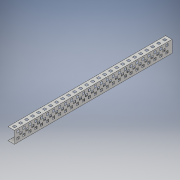
# Autodesk Inventor part: 1sqr x 2sqr x 1sqr metal frame (large)
Saved by Autodesk Inventor 2018 (Build 220112000, 112)
## iProperties
Created: 2018-11-08
Part Number: 1sqr x 2sqr x 1sqr metal frame (large)
Material: Generic
Document SubType Name: Modeling
Designer: USER
Density: 1 g/cm^3
Appearance: Default
Author: USER
Autodesk Inventor part; units mm, degrees
ref_plane "YZ Plane" through (0, 0, 0) normal (1, 0, 0) x (0, 1, 0)
ref_plane "XZ Plane" through (0, 0, 0) normal (0, 1, 0) x (-1, 0, 0)
ref_plane "XY Plane" through (0, 0, 0) normal (0, 0, 1) x (1, 0, 0)
sketch "Sketch1" plane through (0, 0, 0) normal (1, 0, 0) x (0, 1, 0)
  line L0 (0, 0) -> (-24, 0)
  line L1 (-24, 0) -> (-24, -315)
  line L2 (-24, -315) -> (0, -315)
  line L3 (0, -315) -> (0, 0)
  dimension "d0" = 24
  dimension "d1" = 315
  constraints: 8 end point, 2 parallel, 1 horizontal, 1 perpendicular
  measures "d0" distance of L2.end L1.end
  measures "d1" distance of L1.end L0.end
sketch "Sketch2" plane through (0, 0, 0) normal (0, 1, 0) x (-1, 0, 0)
  line L0 (0, 0) -> (13, 0)
  line L1 (13, 0) -> (13, -315)
  line L2 (13, -315) -> (0, -315)
  line L3 (0, -315) -> (0, 0)
  dimension "d2" = 13
  dimension "d3" = 315
  constraints: 8 end point, 2 parallel, 1 horizontal, 1 perpendicular
  measures "d2" distance of L1.end L2.end
  measures "d3" distance of L0.end L1.end
extrude "Extrusion1" add sketch "Sketch2" along normal blind 0.1
extrude "Extrusion2" add sketch "Sketch1" along normal blind 0.1 separate body
sketch "Sketch3" plane through (0, -24, -315) normal (0, -1, 0) x (1, 0, 0)
  line L0 (-13, 315) -> (0, 315) projected
  line L1 (0, 315) -> (-13, 315)
  line L2 (-13, 315) -> (-13, 0)
  line L3 (-13, 0) -> (0, 0)
  line L4 (0, 0) -> (0, 315)
  dimension "d8" = 13
  dimension "d9" = 315
  constraints: 8 end point, 2 parallel, 1 horizontal, 1 perpendicular
  measures "d8" distance of L3.end L2.end
  measures "d9" distance of L2.end L1.end
extrude "Extrusion3" add sketch "Sketch3" along normal blind 0.1 separate body
sketch "Sketch4" plane through (0, 0.1, 0) normal (0, 1, 0) x (1, 0, 0)
  line L0 (-8.9107, 4.7757) -> (-4.3387, 4.7757)
  line L1 (-4.3387, 4.7757) -> (-4.3387, 9.3477)
  line L2 (-4.3387, 9.3477) -> (-8.9107, 9.3477)
  line L3 (-8.9107, 9.3477) -> (-8.9107, 4.7757)
  line L4 (-8.9107, 21.3477) -> (-8.9107, 16.7757)
  line L5 (-8.9107, 16.7757) -> (-4.3387, 16.7757)
  line L6 (-4.3387, 16.7757) -> (-4.3387, 21.3477)
  line L7 (-4.3387, 21.3477) -> (-8.9107, 21.3477)
  line L8 (-8.9107, 33.3477) -> (-8.9107, 28.7757)
  line L9 (-8.9107, 28.7757) -> (-4.3387, 28.7757)
  line L10 (-4.3387, 28.7757) -> (-4.3387, 33.3477)
  line L11 (-4.3387, 33.3477) -> (-8.9107, 33.3477)
  line L12 (-8.9107, 45.3477) -> (-8.9107, 40.7757)
  line L13 (-8.9107, 40.7757) -> (-4.3387, 40.7757)
  line L14 (-4.3387, 40.7757) -> (-4.3387, 45.3477)
  line L15 (-4.3387, 45.3477) -> (-8.9107, 45.3477)
  line L16 (-8.9107, 57.3477) -> (-8.9107, 52.7757)
  line L17 (-8.9107, 52.7757) -> (-4.3387, 52.7757)
  line L18 (-4.3387, 52.7757) -> (-4.3387, 57.3477)
  line L19 (-4.3387, 57.3477) -> (-8.9107, 57.3477)
  line L20 (-8.9107, 69.3477) -> (-8.9107, 64.7757)
  line L21 (-8.9107, 64.7757) -> (-4.3387, 64.7757)
  line L22 (-4.3387, 64.7757) -> (-4.3387, 69.3477)
  line L23 (-4.3387, 69.3477) -> (-8.9107, 69.3477)
  line L24 (-8.9107, 81.3477) -> (-8.9107, 76.7757)
  line L25 (-8.9107, 76.7757) -> (-4.3387, 76.7757)
  line L26 (-4.3387, 76.7757) -> (-4.3387, 81.3477)
  line L27 (-4.3387, 81.3477) -> (-8.9107, 81.3477)
  line L28 (-8.9107, 93.3477) -> (-8.9107, 88.7757)
  line L29 (-8.9107, 88.7757) -> (-4.3387, 88.7757)
  line L30 (-4.3387, 88.7757) -> (-4.3387, 93.3477)
  line L31 (-4.3387, 93.3477) -> (-8.9107, 93.3477)
  line L32 (-8.9107, 105.3477) -> (-8.9107, 100.7757)
  line L33 (-8.9107, 100.7757) -> (-4.3387, 100.7757)
  line L34 (-4.3387, 100.7757) -> (-4.3387, 105.3477)
  line L35 (-4.3387, 105.3477) -> (-8.9107, 105.3477)
  line L36 (-8.9107, 117.3477) -> (-8.9107, 112.7757)
  line L37 (-8.9107, 112.7757) -> (-4.3387, 112.7757)
  line L38 (-4.3387, 112.7757) -> (-4.3387, 117.3477)
  line L39 (-4.3387, 117.3477) -> (-8.9107, 117.3477)
  line L40 (-8.9107, 129.3477) -> (-8.9107, 124.7757)
  line L41 (-8.9107, 124.7757) -> (-4.3387, 124.7757)
  line L42 (-4.3387, 124.7757) -> (-4.3387, 129.3477)
  line L43 (-4.3387, 129.3477) -> (-8.9107, 129.3477)
  line L44 (-8.9107, 141.3477) -> (-8.9107, 136.7757)
  line L45 (-8.9107, 136.7757) -> (-4.3387, 136.7757)
  line L46 (-4.3387, 136.7757) -> (-4.3387, 141.3477)
  line L47 (-4.3387, 141.3477) -> (-8.9107, 141.3477)
  line L48 (-8.9107, 153.3477) -> (-8.9107, 148.7757)
  line L49 (-8.9107, 148.7757) -> (-4.3387, 148.7757)
  line L50 (-4.3387, 148.7757) -> (-4.3387, 153.3477)
  line L51 (-4.3387, 153.3477) -> (-8.9107, 153.3477)
  line L52 (-8.9107, 165.3477) -> (-8.9107, 160.7757)
  line L53 (-8.9107, 160.7757) -> (-4.3387, 160.7757)
  line L54 (-4.3387, 160.7757) -> (-4.3387, 165.3477)
  line L55 (-4.3387, 165.3477) -> (-8.9107, 165.3477)
  line L56 (-8.9107, 177.3477) -> (-8.9107, 172.7757)
  line L57 (-8.9107, 172.7757) -> (-4.3387, 172.7757)
  line L58 (-4.3387, 172.7757) -> (-4.3387, 177.3477)
  line L59 (-4.3387, 177.3477) -> (-8.9107, 177.3477)
  line L60 (-8.9107, 189.3477) -> (-8.9107, 184.7757)
  line L61 (-8.9107, 184.7757) -> (-4.3387, 184.7757)
  line L62 (-4.3387, 184.7757) -> (-4.3387, 189.3477)
  line L63 (-4.3387, 189.3477) -> (-8.9107, 189.3477)
  line L64 (-8.9107, 201.3477) -> (-8.9107, 196.7757)
  line L65 (-8.9107, 196.7757) -> (-4.3387, 196.7757)
  line L66 (-4.3387, 196.7757) -> (-4.3387, 201.3477)
  line L67 (-4.3387, 201.3477) -> (-8.9107, 201.3477)
  line L68 (-8.9107, 213.3477) -> (-8.9107, 208.7757)
  line L69 (-8.9107, 208.7757) -> (-4.3387, 208.7757)
  line L70 (-4.3387, 208.7757) -> (-4.3387, 213.3477)
  line L71 (-4.3387, 213.3477) -> (-8.9107, 213.3477)
  line L72 (-8.9107, 225.3477) -> (-8.9107, 220.7757)
  line L73 (-8.9107, 220.7757) -> (-4.3387, 220.7757)
  line L74 (-4.3387, 220.7757) -> (-4.3387, 225.3477)
  line L75 (-4.3387, 225.3477) -> (-8.9107, 225.3477)
  line L76 (-8.9107, 237.3477) -> (-8.9107, 232.7757)
  line L77 (-8.9107, 232.7757) -> (-4.3387, 232.7757)
  line L78 (-4.3387, 232.7757) -> (-4.3387, 237.3477)
  line L79 (-4.3387, 237.3477) -> (-8.9107, 237.3477)
  line L80 (-8.9107, 249.3477) -> (-8.9107, 244.7757)
  line L81 (-8.9107, 244.7757) -> (-4.3387, 244.7757)
  line L82 (-4.3387, 244.7757) -> (-4.3387, 249.3477)
  line L83 (-4.3387, 249.3477) -> (-8.9107, 249.3477)
  line L84 (-8.9107, 261.3477) -> (-8.9107, 256.7757)
  line L85 (-8.9107, 256.7757) -> (-4.3387, 256.7757)
  line L86 (-4.3387, 256.7757) -> (-4.3387, 261.3477)
  line L87 (-4.3387, 261.3477) -> (-8.9107, 261.3477)
  line L88 (-8.9107, 273.3477) -> (-8.9107, 268.7757)
  line L89 (-8.9107, 268.7757) -> (-4.3387, 268.7757)
  line L90 (-4.3387, 268.7757) -> (-4.3387, 273.3477)
  line L91 (-4.3387, 273.3477) -> (-8.9107, 273.3477)
  line L92 (-8.9107, 285.3477) -> (-8.9107, 280.7757)
  line L93 (-8.9107, 280.7757) -> (-4.3387, 280.7757)
  line L94 (-4.3387, 280.7757) -> (-4.3387, 285.3477)
  line L95 (-4.3387, 285.3477) -> (-8.9107, 285.3477)
  line L96 (-8.9107, 297.3477) -> (-8.9107, 292.7757)
  line L97 (-8.9107, 292.7757) -> (-4.3387, 292.7757)
  line L98 (-4.3387, 292.7757) -> (-4.3387, 297.3477)
  line L99 (-4.3387, 297.3477) -> (-8.9107, 297.3477)
  line L100 (-8.9107, 309.3477) -> (-8.9107, 304.7757)
  line L101 (-8.9107, 304.7757) -> (-4.3387, 304.7757)
  line L102 (-4.3387, 304.7757) -> (-4.3387, 309.3477)
  line L103 (-4.3387, 309.3477) -> (-8.9107, 309.3477)
  point P0 (0, 0)
  dimension "d12" = 4.572
  dimension "d13" = 4.572
  dimension "d19" = 12
  constraints: 208 end point, 2 parallel, 1 collinear, 1 horizontal, 1 perpendicular, 1 vertical, 199 other
  measures "d12" distance of L2.end L1.end
  measures "d13" distance of L1.end L0.end
  measures "d19" distance of L2.end L4.start
extrude "Extrusion4" cut sketch "Sketch4" against normal through all bodies 1
sketch "Sketch5" plane through (0, -24.1, -315) normal (0, -1, 0) x (1, 0, 0)
  line L0 (-8.9107, 305.6523) -> (-4.3387, 305.6523) projected
  line L1 (-8.9107, 305.6523) -> (-4.3387, 305.6523)
  line L2 (-4.3387, 305.6523) -> (-4.3387, 301.0803)
  line L3 (-4.3387, 301.0803) -> (-8.9107, 301.0803)
  line L4 (-8.9107, 301.0803) -> (-8.9107, 305.6523)
  line L5 (-8.9107, 289.1803) -> (-8.9107, 293.7523)
  line L6 (-4.3387, 289.1803) -> (-8.9107, 289.1803)
  line L7 (-4.3387, 293.7523) -> (-4.3387, 289.1803)
  line L8 (-8.9107, 293.7523) -> (-4.3387, 293.7523)
  line L9 (-8.9107, 277.2803) -> (-8.9107, 281.8523)
  line L10 (-4.3387, 277.2803) -> (-8.9107, 277.2803)
  line L11 (-4.3387, 281.8523) -> (-4.3387, 277.2803)
  line L12 (-8.9107, 281.8523) -> (-4.3387, 281.8523)
  line L13 (-8.9107, 265.3803) -> (-8.9107, 269.9523)
  line L14 (-4.3387, 265.3803) -> (-8.9107, 265.3803)
  line L15 (-4.3387, 269.9523) -> (-4.3387, 265.3803)
  line L16 (-8.9107, 269.9523) -> (-4.3387, 269.9523)
  line L17 (-8.9107, 253.4803) -> (-8.9107, 258.0523)
  line L18 (-4.3387, 253.4803) -> (-8.9107, 253.4803)
  line L19 (-4.3387, 258.0523) -> (-4.3387, 253.4803)
  line L20 (-8.9107, 258.0523) -> (-4.3387, 258.0523)
  line L21 (-8.9107, 241.5803) -> (-8.9107, 246.1523)
  line L22 (-4.3387, 241.5803) -> (-8.9107, 241.5803)
  line L23 (-4.3387, 246.1523) -> (-4.3387, 241.5803)
  line L24 (-8.9107, 246.1523) -> (-4.3387, 246.1523)
  line L25 (-8.9107, 229.6803) -> (-8.9107, 234.2523)
  line L26 (-4.3387, 229.6803) -> (-8.9107, 229.6803)
  line L27 (-4.3387, 234.2523) -> (-4.3387, 229.6803)
  line L28 (-8.9107, 234.2523) -> (-4.3387, 234.2523)
  line L29 (-8.9107, 217.7803) -> (-8.9107, 222.3523)
  line L30 (-4.3387, 217.7803) -> (-8.9107, 217.7803)
  line L31 (-4.3387, 222.3523) -> (-4.3387, 217.7803)
  line L32 (-8.9107, 222.3523) -> (-4.3387, 222.3523)
  line L33 (-8.9107, 205.8803) -> (-8.9107, 210.4523)
  line L34 (-4.3387, 205.8803) -> (-8.9107, 205.8803)
  line L35 (-4.3387, 210.4523) -> (-4.3387, 205.8803)
  line L36 (-8.9107, 210.4523) -> (-4.3387, 210.4523)
  line L37 (-8.9107, 193.9803) -> (-8.9107, 198.5523)
  line L38 (-4.3387, 193.9803) -> (-8.9107, 193.9803)
  line L39 (-4.3387, 198.5523) -> (-4.3387, 193.9803)
  line L40 (-8.9107, 198.5523) -> (-4.3387, 198.5523)
  line L41 (-8.9107, 182.0803) -> (-8.9107, 186.6523)
  line L42 (-4.3387, 182.0803) -> (-8.9107, 182.0803)
  line L43 (-4.3387, 186.6523) -> (-4.3387, 182.0803)
  line L44 (-8.9107, 186.6523) -> (-4.3387, 186.6523)
  line L45 (-8.9107, 170.1803) -> (-8.9107, 174.7523)
  line L46 (-4.3387, 170.1803) -> (-8.9107, 170.1803)
  line L47 (-4.3387, 174.7523) -> (-4.3387, 170.1803)
  line L48 (-8.9107, 174.7523) -> (-4.3387, 174.7523)
  line L49 (-8.9107, 158.2803) -> (-8.9107, 162.8523)
  line L50 (-4.3387, 158.2803) -> (-8.9107, 158.2803)
  line L51 (-4.3387, 162.8523) -> (-4.3387, 158.2803)
  line L52 (-8.9107, 162.8523) -> (-4.3387, 162.8523)
  line L53 (-8.9107, 146.3803) -> (-8.9107, 150.9523)
  line L54 (-4.3387, 146.3803) -> (-8.9107, 146.3803)
  line L55 (-4.3387, 150.9523) -> (-4.3387, 146.3803)
  line L56 (-8.9107, 150.9523) -> (-4.3387, 150.9523)
  line L57 (-8.9107, 134.4803) -> (-8.9107, 139.0523)
  line L58 (-4.3387, 134.4803) -> (-8.9107, 134.4803)
  line L59 (-4.3387, 139.0523) -> (-4.3387, 134.4803)
  line L60 (-8.9107, 139.0523) -> (-4.3387, 139.0523)
  line L61 (-8.9107, 122.5803) -> (-8.9107, 127.1523)
  line L62 (-4.3387, 122.5803) -> (-8.9107, 122.5803)
  line L63 (-4.3387, 127.1523) -> (-4.3387, 122.5803)
  line L64 (-8.9107, 127.1523) -> (-4.3387, 127.1523)
  line L65 (-8.9107, 110.6803) -> (-8.9107, 115.2523)
  line L66 (-4.3387, 110.6803) -> (-8.9107, 110.6803)
  line L67 (-4.3387, 115.2523) -> (-4.3387, 110.6803)
  line L68 (-8.9107, 115.2523) -> (-4.3387, 115.2523)
  line L69 (-8.9107, 98.7803) -> (-8.9107, 103.3523)
  line L70 (-4.3387, 98.7803) -> (-8.9107, 98.7803)
  line L71 (-4.3387, 103.3523) -> (-4.3387, 98.7803)
  line L72 (-8.9107, 103.3523) -> (-4.3387, 103.3523)
  line L73 (-8.9107, 86.8803) -> (-8.9107, 91.4523)
  line L74 (-4.3387, 86.8803) -> (-8.9107, 86.8803)
  line L75 (-4.3387, 91.4523) -> (-4.3387, 86.8803)
  line L76 (-8.9107, 91.4523) -> (-4.3387, 91.4523)
  line L77 (-8.9107, 74.9803) -> (-8.9107, 79.5523)
  line L78 (-4.3387, 74.9803) -> (-8.9107, 74.9803)
  line L79 (-4.3387, 79.5523) -> (-4.3387, 74.9803)
  line L80 (-8.9107, 79.5523) -> (-4.3387, 79.5523)
  line L81 (-8.9107, 63.0803) -> (-8.9107, 67.6523)
  line L82 (-4.3387, 63.0803) -> (-8.9107, 63.0803)
  line L83 (-4.3387, 67.6523) -> (-4.3387, 63.0803)
  line L84 (-8.9107, 67.6523) -> (-4.3387, 67.6523)
  line L85 (-8.9107, 51.1803) -> (-8.9107, 55.7523)
  line L86 (-4.3387, 51.1803) -> (-8.9107, 51.1803)
  line L87 (-4.3387, 55.7523) -> (-4.3387, 51.1803)
  line L88 (-8.9107, 55.7523) -> (-4.3387, 55.7523)
  line L89 (-8.9107, 39.2803) -> (-8.9107, 43.8523)
  line L90 (-4.3387, 39.2803) -> (-8.9107, 39.2803)
  line L91 (-4.3387, 43.8523) -> (-4.3387, 39.2803)
  line L92 (-8.9107, 43.8523) -> (-4.3387, 43.8523)
  line L93 (-8.9107, 27.3803) -> (-8.9107, 31.9523)
  line L94 (-4.3387, 27.3803) -> (-8.9107, 27.3803)
  line L95 (-4.3387, 31.9523) -> (-4.3387, 27.3803)
  line L96 (-8.9107, 31.9523) -> (-4.3387, 31.9523)
  line L97 (-8.9107, 15.4803) -> (-8.9107, 20.0523)
  line L98 (-4.3387, 15.4803) -> (-8.9107, 15.4803)
  line L99 (-4.3387, 20.0523) -> (-4.3387, 15.4803)
  line L100 (-8.9107, 20.0523) -> (-4.3387, 20.0523)
  line L101 (-8.9107, 3.5803) -> (-8.9107, 8.1523)
  line L102 (-4.3387, 3.5803) -> (-8.9107, 3.5803)
  line L103 (-4.3387, 8.1523) -> (-4.3387, 3.5803)
  line L104 (-8.9107, 8.1523) -> (-4.3387, 8.1523)
  point P0 (0, 315)
  dimension "d23" = 4.572
  dimension "d29" = 11.9
  constraints: 208 end point, 2 parallel, 1 collinear, 1 horizontal, 1 perpendicular, 1 vertical, 199 other
  measures "d23" distance of L1.end L2.end
  measures "d29" distance of L3.end L5.start
extrude "Extrusion5" cut sketch "Sketch5" against normal through all bodies 3
sketch "Sketch6" plane through (0.1, 0, 0) normal (1, 0, 0) x (0, 0, -1)
  line L0 (4.8427, -2.721) -> (9.4147, -2.721)
  line L1 (9.4147, -2.721) -> (9.4147, -7.293)
  line L2 (9.4147, -7.293) -> (4.8427, -7.293)
  line L3 (4.8427, -7.293) -> (4.8427, -2.721)
  line L4 (16.7427, -2.721) -> (21.3147, -2.721)
  line L5 (16.7427, -7.293) -> (16.7427, -2.721)
  line L6 (21.3147, -7.293) -> (16.7427, -7.293)
  line L7 (21.3147, -2.721) -> (21.3147, -7.293)
  line L8 (28.6427, -2.721) -> (33.2147, -2.721)
  line L9 (28.6427, -7.293) -> (28.6427, -2.721)
  line L10 (33.2147, -7.293) -> (28.6427, -7.293)
  line L11 (33.2147, -2.721) -> (33.2147, -7.293)
  line L12 (40.5427, -2.721) -> (45.1147, -2.721)
  line L13 (40.5427, -7.293) -> (40.5427, -2.721)
  line L14 (45.1147, -7.293) -> (40.5427, -7.293)
  line L15 (45.1147, -2.721) -> (45.1147, -7.293)
  line L16 (52.4427, -2.721) -> (57.0147, -2.721)
  line L17 (52.4427, -7.293) -> (52.4427, -2.721)
  line L18 (57.0147, -7.293) -> (52.4427, -7.293)
  line L19 (57.0147, -2.721) -> (57.0147, -7.293)
  line L20 (64.3427, -2.721) -> (68.9147, -2.721)
  line L21 (64.3427, -7.293) -> (64.3427, -2.721)
  line L22 (68.9147, -7.293) -> (64.3427, -7.293)
  line L23 (68.9147, -2.721) -> (68.9147, -7.293)
  line L24 (76.2427, -2.721) -> (80.8147, -2.721)
  line L25 (76.2427, -7.293) -> (76.2427, -2.721)
  line L26 (80.8147, -7.293) -> (76.2427, -7.293)
  line L27 (80.8147, -2.721) -> (80.8147, -7.293)
  line L28 (88.1427, -2.721) -> (92.7147, -2.721)
  line L29 (88.1427, -7.293) -> (88.1427, -2.721)
  line L30 (92.7147, -7.293) -> (88.1427, -7.293)
  line L31 (92.7147, -2.721) -> (92.7147, -7.293)
  line L32 (100.0427, -2.721) -> (104.6147, -2.721)
  line L33 (100.0427, -7.293) -> (100.0427, -2.721)
  line L34 (104.6147, -7.293) -> (100.0427, -7.293)
  line L35 (104.6147, -2.721) -> (104.6147, -7.293)
  line L36 (111.9427, -2.721) -> (116.5147, -2.721)
  line L37 (111.9427, -7.293) -> (111.9427, -2.721)
  line L38 (116.5147, -7.293) -> (111.9427, -7.293)
  line L39 (116.5147, -2.721) -> (116.5147, -7.293)
  line L40 (123.8427, -2.721) -> (128.4147, -2.721)
  line L41 (123.8427, -7.293) -> (123.8427, -2.721)
  line L42 (128.4147, -7.293) -> (123.8427, -7.293)
  line L43 (128.4147, -2.721) -> (128.4147, -7.293)
  line L44 (135.7427, -2.721) -> (140.3147, -2.721)
  line L45 (135.7427, -7.293) -> (135.7427, -2.721)
  line L46 (140.3147, -7.293) -> (135.7427, -7.293)
  line L47 (140.3147, -2.721) -> (140.3147, -7.293)
  line L48 (147.6427, -2.721) -> (152.2147, -2.721)
  line L49 (147.6427, -7.293) -> (147.6427, -2.721)
  line L50 (152.2147, -7.293) -> (147.6427, -7.293)
  line L51 (152.2147, -2.721) -> (152.2147, -7.293)
  line L52 (159.5427, -2.721) -> (164.1147, -2.721)
  line L53 (159.5427, -7.293) -> (159.5427, -2.721)
  line L54 (164.1147, -7.293) -> (159.5427, -7.293)
  line L55 (164.1147, -2.721) -> (164.1147, -7.293)
  line L56 (171.4427, -2.721) -> (176.0147, -2.721)
  line L57 (171.4427, -7.293) -> (171.4427, -2.721)
  line L58 (176.0147, -7.293) -> (171.4427, -7.293)
  line L59 (176.0147, -2.721) -> (176.0147, -7.293)
  line L60 (183.3427, -2.721) -> (187.9147, -2.721)
  line L61 (183.3427, -7.293) -> (183.3427, -2.721)
  line L62 (187.9147, -7.293) -> (183.3427, -7.293)
  line L63 (187.9147, -2.721) -> (187.9147, -7.293)
  line L64 (195.2427, -2.721) -> (199.8147, -2.721)
  line L65 (195.2427, -7.293) -> (195.2427, -2.721)
  line L66 (199.8147, -7.293) -> (195.2427, -7.293)
  line L67 (199.8147, -2.721) -> (199.8147, -7.293)
  line L68 (207.1427, -2.721) -> (211.7147, -2.721)
  line L69 (207.1427, -7.293) -> (207.1427, -2.721)
  line L70 (211.7147, -7.293) -> (207.1427, -7.293)
  line L71 (211.7147, -2.721) -> (211.7147, -7.293)
  line L72 (219.0427, -2.721) -> (223.6147, -2.721)
  line L73 (219.0427, -7.293) -> (219.0427, -2.721)
  line L74 (223.6147, -7.293) -> (219.0427, -7.293)
  line L75 (223.6147, -2.721) -> (223.6147, -7.293)
  line L76 (230.9427, -2.721) -> (235.5147, -2.721)
  line L77 (230.9427, -7.293) -> (230.9427, -2.721)
  line L78 (235.5147, -7.293) -> (230.9427, -7.293)
  line L79 (235.5147, -2.721) -> (235.5147, -7.293)
  line L80 (242.8427, -2.721) -> (247.4147, -2.721)
  line L81 (242.8427, -7.293) -> (242.8427, -2.721)
  line L82 (247.4147, -7.293) -> (242.8427, -7.293)
  line L83 (247.4147, -2.721) -> (247.4147, -7.293)
  line L84 (254.7427, -2.721) -> (259.3147, -2.721)
  line L85 (254.7427, -7.293) -> (254.7427, -2.721)
  line L86 (259.3147, -7.293) -> (254.7427, -7.293)
  line L87 (259.3147, -2.721) -> (259.3147, -7.293)
  line L88 (266.6427, -2.721) -> (271.2147, -2.721)
  line L89 (266.6427, -7.293) -> (266.6427, -2.721)
  line L90 (271.2147, -7.293) -> (266.6427, -7.293)
  line L91 (271.2147, -2.721) -> (271.2147, -7.293)
  line L92 (278.5427, -2.721) -> (283.1147, -2.721)
  line L93 (278.5427, -7.293) -> (278.5427, -2.721)
  line L94 (283.1147, -7.293) -> (278.5427, -7.293)
  line L95 (283.1147, -2.721) -> (283.1147, -7.293)
  line L96 (290.4427, -2.721) -> (295.0147, -2.721)
  line L97 (290.4427, -7.293) -> (290.4427, -2.721)
  line L98 (295.0147, -7.293) -> (290.4427, -7.293)
  line L99 (295.0147, -2.721) -> (295.0147, -7.293)
  line L100 (302.3427, -2.721) -> (306.9147, -2.721)
  line L101 (302.3427, -7.293) -> (302.3427, -2.721)
  line L102 (306.9147, -7.293) -> (302.3427, -7.293)
  line L103 (306.9147, -2.721) -> (306.9147, -7.293)
  line L104 (4.8427, -14.721) -> (9.4147, -14.721)
  line L105 (4.8427, -19.293) -> (4.8427, -14.721)
  line L106 (9.4147, -19.293) -> (4.8427, -19.293)
  line L107 (9.4147, -14.721) -> (9.4147, -19.293)
  line L108 (16.7427, -14.721) -> (21.3147, -14.721)
  line L109 (16.7427, -19.293) -> (16.7427, -14.721)
  line L110 (21.3147, -19.293) -> (16.7427, -19.293)
  line L111 (21.3147, -14.721) -> (21.3147, -19.293)
  line L112 (28.6427, -14.721) -> (33.2147, -14.721)
  line L113 (28.6427, -19.293) -> (28.6427, -14.721)
  line L114 (33.2147, -19.293) -> (28.6427, -19.293)
  line L115 (33.2147, -14.721) -> (33.2147, -19.293)
  line L116 (40.5427, -14.721) -> (45.1147, -14.721)
  line L117 (40.5427, -19.293) -> (40.5427, -14.721)
  line L118 (45.1147, -19.293) -> (40.5427, -19.293)
  line L119 (45.1147, -14.721) -> (45.1147, -19.293)
  line L120 (52.4427, -14.721) -> (57.0147, -14.721)
  line L121 (52.4427, -19.293) -> (52.4427, -14.721)
  line L122 (57.0147, -19.293) -> (52.4427, -19.293)
  line L123 (57.0147, -14.721) -> (57.0147, -19.293)
  line L124 (64.3427, -14.721) -> (68.9147, -14.721)
  line L125 (64.3427, -19.293) -> (64.3427, -14.721)
  line L126 (68.9147, -19.293) -> (64.3427, -19.293)
  line L127 (68.9147, -14.721) -> (68.9147, -19.293)
  line L128 (76.2427, -14.721) -> (80.8147, -14.721)
  line L129 (76.2427, -19.293) -> (76.2427, -14.721)
  line L130 (80.8147, -19.293) -> (76.2427, -19.293)
  line L131 (80.8147, -14.721) -> (80.8147, -19.293)
  line L132 (88.1427, -14.721) -> (92.7147, -14.721)
  line L133 (88.1427, -19.293) -> (88.1427, -14.721)
  line L134 (92.7147, -19.293) -> (88.1427, -19.293)
  line L135 (92.7147, -14.721) -> (92.7147, -19.293)
  line L136 (100.0427, -14.721) -> (104.6147, -14.721)
  line L137 (100.0427, -19.293) -> (100.0427, -14.721)
  line L138 (104.6147, -19.293) -> (100.0427, -19.293)
  line L139 (104.6147, -14.721) -> (104.6147, -19.293)
  line L140 (111.9427, -14.721) -> (116.5147, -14.721)
  line L141 (111.9427, -19.293) -> (111.9427, -14.721)
  line L142 (116.5147, -19.293) -> (111.9427, -19.293)
  line L143 (116.5147, -14.721) -> (116.5147, -19.293)
  line L144 (123.8427, -14.721) -> (128.4147, -14.721)
  line L145 (123.8427, -19.293) -> (123.8427, -14.721)
  line L146 (128.4147, -19.293) -> (123.8427, -19.293)
  line L147 (128.4147, -14.721) -> (128.4147, -19.293)
  line L148 (135.7427, -14.721) -> (140.3147, -14.721)
  line L149 (135.7427, -19.293) -> (135.7427, -14.721)
  line L150 (140.3147, -19.293) -> (135.7427, -19.293)
  line L151 (140.3147, -14.721) -> (140.3147, -19.293)
  line L152 (147.6427, -14.721) -> (152.2147, -14.721)
  line L153 (147.6427, -19.293) -> (147.6427, -14.721)
  line L154 (152.2147, -19.293) -> (147.6427, -19.293)
  line L155 (152.2147, -14.721) -> (152.2147, -19.293)
  line L156 (159.5427, -14.721) -> (164.1147, -14.721)
  line L157 (159.5427, -19.293) -> (159.5427, -14.721)
  line L158 (164.1147, -19.293) -> (159.5427, -19.293)
  line L159 (164.1147, -14.721) -> (164.1147, -19.293)
  line L160 (171.4427, -14.721) -> (176.0147, -14.721)
  line L161 (171.4427, -19.293) -> (171.4427, -14.721)
  line L162 (176.0147, -19.293) -> (171.4427, -19.293)
  line L163 (176.0147, -14.721) -> (176.0147, -19.293)
  line L164 (183.3427, -14.721) -> (187.9147, -14.721)
  line L165 (183.3427, -19.293) -> (183.3427, -14.721)
  line L166 (187.9147, -19.293) -> (183.3427, -19.293)
  line L167 (187.9147, -14.721) -> (187.9147, -19.293)
  line L168 (195.2427, -14.721) -> (199.8147, -14.721)
  line L169 (195.2427, -19.293) -> (195.2427, -14.721)
  line L170 (199.8147, -19.293) -> (195.2427, -19.293)
  line L171 (199.8147, -14.721) -> (199.8147, -19.293)
  line L172 (207.1427, -14.721) -> (211.7147, -14.721)
  line L173 (207.1427, -19.293) -> (207.1427, -14.721)
  line L174 (211.7147, -19.293) -> (207.1427, -19.293)
  line L175 (211.7147, -14.721) -> (211.7147, -19.293)
  line L176 (219.0427, -14.721) -> (223.6147, -14.721)
  line L177 (219.0427, -19.293) -> (219.0427, -14.721)
  line L178 (223.6147, -19.293) -> (219.0427, -19.293)
  line L179 (223.6147, -14.721) -> (223.6147, -19.293)
  line L180 (230.9427, -14.721) -> (235.5147, -14.721)
  line L181 (230.9427, -19.293) -> (230.9427, -14.721)
  line L182 (235.5147, -19.293) -> (230.9427, -19.293)
  line L183 (235.5147, -14.721) -> (235.5147, -19.293)
  line L184 (242.8427, -14.721) -> (247.4147, -14.721)
  line L185 (242.8427, -19.293) -> (242.8427, -14.721)
  line L186 (247.4147, -19.293) -> (242.8427, -19.293)
  line L187 (247.4147, -14.721) -> (247.4147, -19.293)
  line L188 (254.7427, -14.721) -> (259.3147, -14.721)
  line L189 (254.7427, -19.293) -> (254.7427, -14.721)
  line L190 (259.3147, -19.293) -> (254.7427, -19.293)
  line L191 (259.3147, -14.721) -> (259.3147, -19.293)
  line L192 (266.6427, -14.721) -> (271.2147, -14.721)
  line L193 (266.6427, -19.293) -> (266.6427, -14.721)
  line L194 (271.2147, -19.293) -> (266.6427, -19.293)
  line L195 (271.2147, -14.721) -> (271.2147, -19.293)
  line L196 (278.5427, -14.721) -> (283.1147, -14.721)
  line L197 (278.5427, -19.293) -> (278.5427, -14.721)
  line L198 (283.1147, -19.293) -> (278.5427, -19.293)
  line L199 (283.1147, -14.721) -> (283.1147, -19.293)
  line L200 (290.4427, -14.721) -> (295.0147, -14.721)
  line L201 (290.4427, -19.293) -> (290.4427, -14.721)
  line L202 (295.0147, -19.293) -> (290.4427, -19.293)
  line L203 (295.0147, -14.721) -> (295.0147, -19.293)
  line L204 (302.3427, -14.721) -> (306.9147, -14.721)
  line L205 (302.3427, -19.293) -> (302.3427, -14.721)
  line L206 (306.9147, -19.293) -> (302.3427, -19.293)
  line L207 (306.9147, -14.721) -> (306.9147, -19.293)
  line L208 (10.732, -8.4176) -> (15.304, -8.4176)
  line L209 (15.304, -8.4176) -> (15.304, -12.9896)
  line L210 (15.304, -12.9896) -> (10.732, -12.9896)
  line L211 (10.732, -12.9896) -> (10.732, -8.4176)
  line L212 (22.632, -8.4176) -> (27.204, -8.4176)
  line L213 (22.632, -12.9896) -> (22.632, -8.4176)
  line L214 (27.204, -8.4176) -> (27.204, -12.9896)
  line L215 (27.204, -12.9896) -> (22.632, -12.9896)
  line L216 (34.532, -8.4176) -> (39.104, -8.4176)
  line L217 (34.532, -12.9896) -> (34.532, -8.4176)
  line L218 (39.104, -8.4176) -> (39.104, -12.9896)
  line L219 (39.104, -12.9896) -> (34.532, -12.9896)
  line L220 (46.432, -8.4176) -> (51.004, -8.4176)
  line L221 (46.432, -12.9896) -> (46.432, -8.4176)
  line L222 (51.004, -8.4176) -> (51.004, -12.9896)
  line L223 (51.004, -12.9896) -> (46.432, -12.9896)
  line L224 (58.332, -8.4176) -> (62.904, -8.4176)
  line L225 (58.332, -12.9896) -> (58.332, -8.4176)
  line L226 (62.904, -8.4176) -> (62.904, -12.9896)
  line L227 (62.904, -12.9896) -> (58.332, -12.9896)
  line L228 (70.232, -8.4176) -> (74.804, -8.4176)
  line L229 (70.232, -12.9896) -> (70.232, -8.4176)
  line L230 (74.804, -8.4176) -> (74.804, -12.9896)
  line L231 (74.804, -12.9896) -> (70.232, -12.9896)
  line L232 (82.132, -8.4176) -> (86.704, -8.4176)
  line L233 (82.132, -12.9896) -> (82.132, -8.4176)
  line L234 (86.704, -8.4176) -> (86.704, -12.9896)
  line L235 (86.704, -12.9896) -> (82.132, -12.9896)
  line L236 (94.032, -8.4176) -> (98.604, -8.4176)
  line L237 (94.032, -12.9896) -> (94.032, -8.4176)
  line L238 (98.604, -8.4176) -> (98.604, -12.9896)
  line L239 (98.604, -12.9896) -> (94.032, -12.9896)
  line L240 (105.932, -8.4176) -> (110.504, -8.4176)
  line L241 (105.932, -12.9896) -> (105.932, -8.4176)
  line L242 (110.504, -8.4176) -> (110.504, -12.9896)
  line L243 (110.504, -12.9896) -> (105.932, -12.9896)
  line L244 (117.832, -8.4176) -> (122.404, -8.4176)
  line L245 (117.832, -12.9896) -> (117.832, -8.4176)
  line L246 (122.404, -8.4176) -> (122.404, -12.9896)
  line L247 (122.404, -12.9896) -> (117.832, -12.9896)
  line L248 (129.732, -8.4176) -> (134.304, -8.4176)
  line L249 (129.732, -12.9896) -> (129.732, -8.4176)
  line L250 (134.304, -8.4176) -> (134.304, -12.9896)
  line L251 (134.304, -12.9896) -> (129.732, -12.9896)
  line L252 (141.632, -8.4176) -> (146.204, -8.4176)
  line L253 (141.632, -12.9896) -> (141.632, -8.4176)
  line L254 (146.204, -8.4176) -> (146.204, -12.9896)
  line L255 (146.204, -12.9896) -> (141.632, -12.9896)
  line L256 (153.532, -8.4176) -> (158.104, -8.4176)
  line L257 (153.532, -12.9896) -> (153.532, -8.4176)
  line L258 (158.104, -8.4176) -> (158.104, -12.9896)
  line L259 (158.104, -12.9896) -> (153.532, -12.9896)
  line L260 (165.432, -8.4176) -> (170.004, -8.4176)
  line L261 (165.432, -12.9896) -> (165.432, -8.4176)
  line L262 (170.004, -8.4176) -> (170.004, -12.9896)
  line L263 (170.004, -12.9896) -> (165.432, -12.9896)
  line L264 (177.332, -8.4176) -> (181.904, -8.4176)
  line L265 (177.332, -12.9896) -> (177.332, -8.4176)
  line L266 (181.904, -8.4176) -> (181.904, -12.9896)
  line L267 (181.904, -12.9896) -> (177.332, -12.9896)
  line L268 (189.232, -8.4176) -> (193.804, -8.4176)
  line L269 (189.232, -12.9896) -> (189.232, -8.4176)
  line L270 (193.804, -8.4176) -> (193.804, -12.9896)
  line L271 (193.804, -12.9896) -> (189.232, -12.9896)
  line L272 (201.132, -8.4176) -> (205.704, -8.4176)
  line L273 (201.132, -12.9896) -> (201.132, -8.4176)
  line L274 (205.704, -8.4176) -> (205.704, -12.9896)
  line L275 (205.704, -12.9896) -> (201.132, -12.9896)
  line L276 (213.032, -8.4176) -> (217.604, -8.4176)
  line L277 (213.032, -12.9896) -> (213.032, -8.4176)
  line L278 (217.604, -8.4176) -> (217.604, -12.9896)
  line L279 (217.604, -12.9896) -> (213.032, -12.9896)
  line L280 (224.932, -8.4176) -> (229.504, -8.4176)
  line L281 (224.932, -12.9896) -> (224.932, -8.4176)
  line L282 (229.504, -8.4176) -> (229.504, -12.9896)
  line L283 (229.504, -12.9896) -> (224.932, -12.9896)
  line L284 (236.832, -8.4176) -> (241.404, -8.4176)
  line L285 (236.832, -12.9896) -> (236.832, -8.4176)
  line L286 (241.404, -8.4176) -> (241.404, -12.9896)
  line L287 (241.404, -12.9896) -> (236.832, -12.9896)
  line L288 (248.732, -8.4176) -> (253.304, -8.4176)
  line L289 (248.732, -12.9896) -> (248.732, -8.4176)
  line L290 (253.304, -8.4176) -> (253.304, -12.9896)
  line L291 (253.304, -12.9896) -> (248.732, -12.9896)
  line L292 (260.632, -8.4176) -> (265.204, -8.4176)
  line L293 (260.632, -12.9896) -> (260.632, -8.4176)
  line L294 (265.204, -8.4176) -> (265.204, -12.9896)
  line L295 (265.204, -12.9896) -> (260.632, -12.9896)
  line L296 (272.532, -8.4176) -> (277.104, -8.4176)
  line L297 (272.532, -12.9896) -> (272.532, -8.4176)
  line L298 (277.104, -8.4176) -> (277.104, -12.9896)
  line L299 (277.104, -12.9896) -> (272.532, -12.9896)
  line L300 (284.432, -8.4176) -> (289.004, -8.4176)
  line L301 (284.432, -12.9896) -> (284.432, -8.4176)
  line L302 (289.004, -8.4176) -> (289.004, -12.9896)
  line L303 (289.004, -12.9896) -> (284.432, -12.9896)
  line L304 (296.332, -8.4176) -> (300.904, -8.4176)
  line L305 (296.332, -12.9896) -> (296.332, -8.4176)
  line L306 (300.904, -8.4176) -> (300.904, -12.9896)
  line L307 (300.904, -12.9896) -> (296.332, -12.9896)
  point P0 (0, 0)
  dimension "d33" = 4.572
  dimension "d34" = 4.572
  dimension "d37" = 11.9
  dimension "d40" = 12
  dimension "d43" = 4.572
  dimension "d44" = 4.572
  dimension "d47" = 11.9
  constraints: 616 end point, 4 horizontal, 4 parallel, 3 collinear, 2 perpendicular, 1 vertical, 597 other
  measures "d33" distance of L1.end L2.end
  measures "d34" distance of L0.end L1.end
  measures "d37" distance of L0.start L4.start
  measures "d40" distance of L0.start L104.start
  measures "d43" distance of L209.end L210.end
  measures "d44" distance of L208.end L209.end
  measures "d47" distance of L208.start L212.start
extrude "Extrusion6" cut sketch "Sketch6" against normal through all bodies 2
body "Solid1"
body "Solid2"
body "Solid3"
